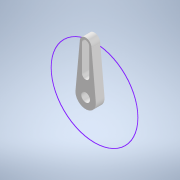
# Autodesk Inventor part: shatun_lidar
Saved by Autodesk Inventor 2022 (Build 260153000, 153)
## iProperties
Created: 2024-10-20
Part Number: shatun_lidar
Material: Типовые
Document SubType Name: Modeling
Designer: Andrey
Density: 1 g/cm^3
Appearance: По умолчанию
Author: Andrey
Autodesk Inventor part; units mm, degrees
ref_plane "YZ Plane" through (0, 0, 0) normal (1, 0, 0) x (0, 1, 0)
ref_plane "XZ Plane" through (0, 0, 0) normal (0, 1, 0) x (-1, 0, 0)
ref_plane "XY Plane" through (0, 0, 0) normal (0, 0, 1) x (1, 0, 0)
sketch "Эскиз1" plane through (0, 0, 0) normal (0, 0, 1) x (1, 0, 0)
  circle A0 centre (0, 0) radius 4 projected
  arc A1 (-13.2, 4.5) -> (-13.2, -4.5) centre (-13.2, 0) ccw projected
  line L0 (-13.2, -4.5) -> (1.3, -4.5) projected
  arc A2 (1.3, -4.5) -> (1.3, 4.5) centre (1.3, 0) ccw projected
  line L1 (1.3, 4.5) -> (-13.2, 4.5) projected
  circle A3 centre (0, 6.5601) radius 1.1 projected
  arc A4 (-6.2548, 22.0866) -> (6.2548, 22.0866) centre (0, 35.5) ccw projected
  arc A5 (7.7339, 18.9146) -> (6.2548, 22.0866) centre (6.9943, 20.5006) ccw projected
  arc A6 (-7.7339, 18.9146) -> (7.7339, 18.9146) centre (0, 35.5) ccw projected
  arc A7 (-6.2548, 22.0866) -> (-7.7339, 18.9146) centre (-6.9943, 20.5006) ccw projected
  line L2 (13.75, 27.1) -> (13.75, 10.8) projected
  line L3 (13.75, 27.1) -> (-13.75, 27.1) projected
  line L4 (-13.75, 27.1) -> (-13.75, 10.8) projected
  line L5 (-13.75, 10.8) -> (-0.7414, 4.9199) projected
  arc A8 (-0.7414, 4.9199) -> (0.7414, 4.9199) centre (0, 6.5601) ccw projected
  line L6 (0.7414, 4.9199) -> (13.75, 10.8) projected
  circle A9 centre (0, 0) radius 12.9209 projected
  circle A10 centre (0, 0) radius 14.9209
  circle A11 centre (-9.898, 8.3054) radius 1.1 projected
  circle A12 centre (-9.898, 8.3054) radius 2
  circle A13 centre (0, 0) radius 1.5
  circle A14 centre (0, 0) radius 3.5
  line L7 (0, 75.6487) -> (0, -4.6487) projected
  line L8 (-1.991, 16.0319) -> (-3.4843, 0.3314)
  line L9 (3.4843, 0.3314) -> (1.991, 16.0319)
  circle A15 centre (0, 6.5601) radius 1.25
  line L10 (1.25, 15.8425) -> (1.25, 6.5601)
  line L11 (-1.25, 6.5601) -> (-1.25, 15.8425)
  arc A16 (14.6884, 10.9864) -> (-14.6884, 10.9864) centre (0, 0) ccw projected
  arc A17 (14.2499, 7.5383) -> (14.6884, 10.9864) centre (12.6864, 9.489) ccw projected
  arc A18 (-14.6884, 10.9864) -> (-14.2594, 7.5459) centre (-12.6864, 9.489) ccw projected
  circle A19 centre (0, 0) radius 15.8425
  circle A20 centre (0, 15.8425) radius 1.25
  circle A21 centre (0, 15.8425) radius 2
  point P0 (0, 0)
  point P1 (-1.25, 12.8603)
  point P2 (1.25, 12.8603)
  point P3 (-1.25, 15.7932)
  point P4 (-1.249, 15.7932)
  point P5 (1.249, 15.7932)
  point P6 (1.25, 15.7932)
  point P7 (2.0213, 15.7131)
  point P8 (1.996, 15.7163)
  point P9 (-1.996, 15.7163)
  point P10 (-2.0213, 15.7131)
  dimension "d0" = 4
  dimension "d1" = 3
  dimension "d2" = 7
  dimension "d6" = 2.5
  dimension "d7" = 2.5
  dimension "d8" = 4
  constraints: 10 point on circle, 9 tangent, 8 centre point, 8 end point, 7 coincident, 1 point on line
  measures "d0" diameter of A12
  measures "d1" diameter of A13
  measures "d2" diameter of A14
  measures "d6" diameter of A15
  measures "d7" diameter of A20
  measures "d8" diameter of A21
extrude "Выдавливание1" add sketch "Эскиз1" along normal blind 3 contours L9 A14 L7 A0 | A0 L7 L1 A2 L9 | L7 A14 L8 A0 | A0 L8 L1 L7 | A14 L7 A13 | A2 L1 L7 A8 L6 L9 | A14 L7 A13 | L1 L8 L5 A8 L7 | L6 A8 L7 A15 L10 A9 L9 | A8 L5 L8 A9 L11 A15 L7 | A9 L10 A21 A10 L9 | A10 A21 A19 L9 | L8 A10 A21 L11 A9 | L10 A10 A21 | A10 L10 A19 A21 | L8 A19 A21 A10 | A19 L10 A20 L7 A6 A21 | A21 A10 L11 | A21 A19 L11 A10 | A6 L7 A21 | A21 A6 L7 A20 L11 A19 | A6 A21 L7 picked at (0.3204, 3.7943) picked at (-0.3204, 3.7943)
sketch "Эскиз2" plane through (0, 0, 0) normal (0, 0, -1) x (-1, 0, 0)
  line L0 (-1.25, 15.7932) -> (-1.25, 6.5601) projected
  line L1 (1.25, 6.5601) -> (1.25, 15.7932) projected
  arc A0 (-1.25, 6.5601) -> (1.25, 6.5601) centre (0, 6.5601) ccw projected
  circle A1 centre (0, 0) radius 14.9209
  arc A2 (1.9865, 13.1531) -> (-1.9865, 13.1531) centre (0, 12.9209) ccw projected
  arc A3 (-1.249, 15.7932) -> (-1.25, 15.7932) centre (0, 0) ccw projected
  arc A4 (1.249, 15.7932) -> (-1.249, 15.7932) centre (0, 15.8425) ccw projected
  arc A5 (1.25, 15.7932) -> (1.249, 15.7932) centre (0, 0) ccw projected
  point P0 (0, 0)
  constraints: 1 centre point, 1 tangent
